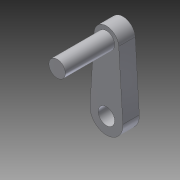
# Autodesk Inventor part: Crank Handle
Saved by Autodesk Inventor 2016 (Build 200138000, 138)
## iProperties
Created: 2014-03-04
Part Number: Crank Handle
Material: PPS Plastic
Document SubType Name: Modeling
Designer: John
Density: 1.637 g/cm^3
Appearance: Smooth - White
Mass: 4.62693 g
Surface Area: 17.5181 cm^2
Volume: 2.82647 cm^3
Author: John
Autodesk Inventor part; units mm, degrees
ref_plane "YZ Plane" through (0, 0, 0) normal (1, 0, 0) x (0, 1, 0)
ref_plane "XZ Plane" through (0, 0, 0) normal (0, 1, 0) x (-1, 0, 0)
ref_plane "XY Plane" through (0, 0, 0) normal (0, 0, 1) x (1, 0, 0)
sketch "Sketch1" plane through (0, 0, 0) normal (0, 0, 1) x (1, 0, 0)
  circle A0 centre (0, 0) radius 6.35
  circle A1 centre (0, 25.4) radius 4.7625
  line L0 (0, 25.4) -> (0, 0)
  line L1 (-4.7532, 25.6977) -> (-6.3376, 0.3969)
  line L2 (6.3376, 0.3969) -> (4.7532, 25.6977)
  dimension "d0" = 12.7
  dimension "d1" = 9.525
  dimension "d2" = 25.4
  constraints: 6 end point, 4 point on circle, 4 tangent, 2 centre point, 1 coincident, 1 vertical
  measures "d0" diameter of A0
  measures "d1" diameter of A1
  measures "d2" distance of L0.start L0.end
extrude "Extrusion1" add sketch "Sketch1" along normal blind 6.35
sketch "Sketch2" plane through (0, 0, 6.35) normal (0, 0, 1) x (1, 0, 0)
  arc A0 (-6.3376, 0.3969) -> (6.3376, 0.3969) centre (0, 0) ccw projected
  circle A1 centre (0, 0) radius 3.175
  dimension "d5" = 6.35
  constraints: 1 centre point, 1 coincident
  measures "d5" diameter of A1
extrude "Extrusion2" cut sketch "Sketch2" against normal through all
sketch "Sketch3" plane through (0, 0, 6.35) normal (0, 0, 1) x (1, 0, 0)
  arc A0 (4.7532, 25.6977) -> (-4.7532, 25.6977) centre (0, 25.4) ccw projected
  circle A1 centre (0, 25.4) radius 3.175
  dimension "d8" = 6.35
  constraints: 1 centre point, 1 coincident
  measures "d8" diameter of A1
extrude "Extrusion3" add sketch "Sketch3" along normal blind 19.05
body "Solid1"
